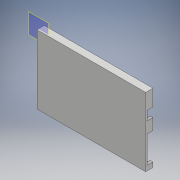
# Autodesk Inventor part: BASE_revised
Saved by Autodesk Inventor 2019 (Build 230136000, 136)
## iProperties
Part Number: BASE_revised
Material: 一般
Document SubType Name: Modeling
Designer: KazutoDell
Density: 1 g/cm^3
Appearance: 既定
Author: KazutoDell
Autodesk Inventor part; units mm, degrees
ref_plane "YZ Plane" through (0, 0, 0) normal (1, 0, 0) x (0, 1, 0)
ref_plane "XZ Plane" through (0, 0, 0) normal (0, 1, 0) x (-1, 0, 0)
ref_plane "XY Plane" through (0, 0, 0) normal (0, 0, 1) x (1, 0, 0)
ref_plane "作業平面1" through (0, 2, 0) normal (0, 1, 0) x (1, 0, 0)
sketch "スケッチ4" plane through (0, 2, 0) normal (0, 1, 0) x (1, 0, 0)
  line L0 (3, 73) -> (33, 73)
  line L1 (3, 73) -> (3, 23)
  line L2 (3, 20) -> (3, 3)
  line L3 (81, 3) -> (81, 33)
  line L4 (81, 33) -> (84, 33)
  line L5 (84, 33) -> (84, 3)
  line L6 (117, 3) -> (117, 18)
  line L7 (117, 18) -> (120, 18)
  line L8 (117, 28) -> (117, 35)
  line L9 (120, 28) -> (117, 28)
  line L10 (120, 28) -> (120, 38)
  line L11 (117, 38) -> (97, 38)
  line L12 (97, 38) -> (97, 45)
  line L13 (97, 45) -> (94, 45)
  line L14 (94, 45) -> (94, 35)
  line L15 (94, 35) -> (117, 35)
  line L16 (97, 73) -> (97, 66)
  line L17 (97, 66) -> (94, 66)
  line L18 (94, 66) -> (94, 73)
  line L19 (33, 73) -> (33, 23)
  line L20 (33, 23) -> (13, 23)
  line L21 (13, 23) -> (13, 20)
  line L22 (13, 20) -> (36, 20)
  line L23 (36, 20) -> (36, 73)
  line L24 (36, 73) -> (46, 73)
  line L25 (46, 73) -> (46, 20)
  line L26 (46, 20) -> (49, 20)
  line L27 (49, 20) -> (49, 73)
  line L28 (117, 38) -> (117, 40.5)
  line L29 (117, 40.5) -> (120, 40.5)
  line L30 (120, 40.5) -> (120, 38)
  line L31 (117, 73) -> (117, 70.5)
  line L32 (117, 70.5) -> (120, 70.5)
  line L33 (0, 0) -> (0, 76)
  line L34 (0, 76) -> (120, 76)
  line L35 (120, 76) -> (120, 70.5)
  line L36 (0, 0) -> (120, 0)
  line L37 (120, 0) -> (120, 18)
  line L38 (3, 23) -> (3, 20)
  line L39 (33, 3) -> (33, 11)
  line L40 (33, 11) -> (36, 11)
  line L41 (36, 11) -> (36, 3)
  line L42 (3, 3) -> (33, 3)
  line L43 (36, 3) -> (81, 3)
  line L44 (94, 3) -> (94, 13)
  line L45 (94, 13) -> (97, 13)
  line L46 (97, 13) -> (97, 3)
  line L47 (84, 3) -> (94, 3)
  line L48 (97, 3) -> (117, 3)
  line L49 (117, 73) -> (97, 73)
  line L50 (94, 73) -> (49, 73)
  dimension "d29" = 3
  dimension "d30" = 30
  dimension "d34" = 3
  dimension "d35" = 20
  dimension "d36" = 3
  dimension "d37" = 10
  dimension "d39" = 3
  dimension "d41" = 32
  dimension "d42" = 3
  dimension "d60" = 3
  dimension "d61" = 3
  dimension "d63" = 7
  dimension "d64" = 7
  dimension "d65" = 15
  dimension "d66" = 10
  dimension "d67" = 2.5
  dimension "d68" = 3
  dimension "d69" = 3
  dimension "d70" = 2.5
  dimension "d75" = 76
  dimension "d78" = 3
  dimension "d79" = 3
  dimension "d80" = 3
  dimension "d81" = 20
  dimension "d82" = 50
  dimension "d84" = 120
  dimension "d85" = 3
  dimension "d86" = 8
  dimension "d87" = 3
  dimension "d88" = 30
  dimension "d89" = 3
  dimension "d90" = 10
  dimension "d91" = 10
  dimension "d92" = 35
  constraints: 103 end point, 31 perpendicular, 15 collinear, 9 vertical, 4 horizontal, 2 point on line, 1 coincident
  measures "d29" distance between parallel lines of L10 L8
  measures "d30" distance between parallel lines of L19 L1
  measures "d34" distance between parallel lines of L22 L20
  measures "d35" distance of L19.end L20.end
  measures "d36" distance between parallel lines of L19 L23
  measures "d37" distance of L24.end L23.end
  measures "d39" distance between parallel lines of L27 L25
  measures "d41" distance between parallel lines of L27 L3
  measures "d42" distance between parallel lines of L5 L3
  measures "d60" distance between parallel lines of L12 L14
  measures "d61" distance between parallel lines of L15 L11
  measures "d63" distance of L11.end L12.end
  measures "d64" distance of L16.start L16.end
  measures "d65" distance of L6.start L6.end
  measures "d66" distance between parallel lines of L7 L9
  measures "d67" distance of L11.start L28.end
  measures "d68" distance of L28.end L29.end
  measures "d69" distance of L31.end L32.end
  measures "d70" distance of L31.start L31.end
  measures "d75" distance of L33.start L33.end
  measures "d78" distance between parallel lines of L33 L1
  measures "d79" distance between parallel lines of L34 L0
  measures "d80" distance between parallel lines of L6 L37
  measures "d81" distance of L31.start L16.start
  measures "d82" distance of L0.end L19.end
  measures "d84" distance of L33.end L34.end
  measures "d85" distance between parallel lines of L42 L36
  measures "d86" distance of L39.start L39.end
  measures "d87" distance of L39.end L40.end
  measures "d88" distance of L3.start L3.end
  measures "d89" distance of L44.end L45.end
  measures "d90" distance of L44.start L44.end
  measures "d91" distance between parallel lines of L5 L44
  measures "d92" distance between parallel lines of L49 L11
extrude "押し出し5" add sketch "スケッチ4" along normal blind 5
sketch "スケッチ6" plane through (0, 2, 0) normal (0, 1, 0) x (1, 0, 0)
  line L0 (0, 0) -> (120, 0) projected
  line L1 (0, 0) -> (120, 0)
  line L2 (120, 18) -> (117, 18) projected
  line L3 (120, 0) -> (120, 18)
  line L4 (120, 18) -> (117, 18)
  line L5 (117, 18) -> (117, 3) projected
  line L6 (117, 18) -> (117, 3)
  line L7 (3, 3) -> (3, 73) projected
  line L8 (117, 3) -> (3, 3)
  line L9 (3, 3) -> (3, 73)
  line L10 (97, 73) -> (117, 73) projected
  line L11 (3, 73) -> (117, 73)
  line L12 (117, 73) -> (117, 70.5) projected
  line L13 (117, 73) -> (117, 70.5)
  line L14 (117, 70.5) -> (120, 70.5) projected
  line L15 (117, 70.5) -> (120, 70.5)
  line L16 (120, 70.5) -> (120, 76) projected
  line L17 (120, 70.5) -> (120, 76)
  line L18 (120, 76) -> (0, 76) projected
  line L19 (120, 76) -> (0, 76)
  line L20 (0, 76) -> (0, 0) projected
  line L21 (0, 76) -> (0, 0)
  line L22 (120, 28) -> (117, 28) projected
  line L23 (117, 28) -> (120, 28)
  line L24 (120, 40.5) -> (120, 28) projected
  line L25 (120, 28) -> (120, 40.5)
  line L26 (117, 40.5) -> (120, 40.5) projected
  line L27 (120, 40.5) -> (117, 40.5)
  line L28 (117, 40.5) -> (117, 28)
  constraints: 32 end point, 9 collinear, 6 perpendicular, 1 horizontal
extrude "押し出し6" add sketch "スケッチ6" along normal blind 6.5
sketch "スケッチ7" plane through (0, 2, 0) normal (0, 1, 0) x (1, 0, 0)
  line L0 (0, 0) -> (120, 0) projected
  line L1 (120, 70.5) -> (120, 76) projected
  line L2 (0, 0) -> (120, 0)
  line L3 (120, 0) -> (120, 76)
  line L4 (120, 76) -> (0, 76)
  line L5 (0, 76) -> (0, 0)
  constraints: 8 end point, 2 parallel, 1 horizontal, 1 perpendicular
extrude "押し出し7" add sketch "スケッチ7" against normal blind 1.5
